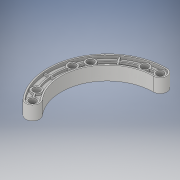
# Autodesk Inventor part: Curved_beam_6h
Saved by Autodesk Inventor 2019 (Build 230136000, 136)
## iProperties
Created: 2019-01-29
Part Number: Curved_beam_6h
Material: Generic
Document SubType Name: Modeling
Designer: Varga Daniel
Density: 1 g/cm^3
Appearance: Default
Author: Varga Daniel
Autodesk Inventor part; units mm, degrees
ref_plane "YZ Plane" through (0, 0, 0) normal (1, 0, 0) x (0, 1, 0)
ref_plane "XZ Plane" through (0, 0, 0) normal (0, 1, 0) x (-1, 0, 0)
ref_plane "XY Plane" through (0, 0, 0) normal (0, 0, 1) x (1, 0, 0)
derived "Base_part.ipt"
sketch "Sketch1" plane through (0, 0, 0) normal (0, 1, 0) x (-1, 0, 0)
  line L0 (5, 0) -> (25, 0)
  line L1 (30, 5) -> (30, 25)
  line L2 (25, 30) -> (5, 30)
  line L3 (0, 25) -> (0, 5)
  line L4 (5, 29) -> (25, 29)
  line L5 (29, 25) -> (29, 5)
  line L6 (25, 1) -> (5, 1)
  line L7 (1, 5) -> (1, 25)
  circle A0 centre (5, 5) radius 2.5
  circle A1 centre (5, 5) radius 3.5
  arc A2 (25, 0) -> (30, 5) centre (25, 5) ccw
  arc A3 (30, 25) -> (25, 30) centre (25, 25) ccw
  arc A4 (5, 30) -> (0, 25) centre (5, 25) ccw
  arc A5 (0, 5) -> (5, 0) centre (5, 5) ccw
  arc A6 (1, 5) -> (5, 1) centre (5, 5) ccw
  arc A7 (5, 29) -> (1, 25) centre (5, 25) ccw
  arc A8 (29, 25) -> (25, 29) centre (25, 25) ccw
  arc A9 (25, 1) -> (29, 5) centre (25, 5) ccw
  line L8 (49.1041, 15) -> (-27.081, 15) construction
  circle A10 centre (5, 15) radius 2.5
  circle A11 centre (5, 15) radius 3.5
  circle A12 centre (15, 5) radius 2.5
  circle A13 centre (15, 5) radius 3.5
  circle A14 centre (15, 15) radius 2.5
  circle A15 centre (15, 15) radius 3.5
  line L9 (1, 9.5) -> (1, 10.5)
  line L10 (29, 10.5) -> (29, 9.5)
  line L11 (31.1478, 10) -> (-2.4877, 10) construction
  line L12 (-2.8604, 5) -> (35.495, 5) construction
  line L13 (11.5359, 5.5) -> (8.4641, 5.5)
  line L14 (11.5359, 4.5) -> (8.4641, 4.5)
  line L15 (5, -2.5736) -> (5, 36.7522) construction
  line L16 (5.5, 8.4641) -> (5.5, 11.5359)
  line L17 (4.5, 8.4641) -> (4.5, 11.5359)
  line L18 (8.4641, 15.5) -> (11.5359, 15.5)
  line L19 (11.5359, 14.5) -> (8.4641, 14.5)
  line L20 (5.5, 1.5359) -> (5.5, 1)
  line L21 (4.5, 1.5359) -> (4.5, 1.0314)
  line L22 (1.5359, 4.5) -> (1.0314, 4.5)
  line L23 (1.5359, 5.5) -> (1, 5.5)
  line L24 (15, -1.4978) -> (15, 34.8784) construction
  line L25 (15.5, 8.4641) -> (15.5, 11.5359)
  line L26 (14.5, 11.5359) -> (14.5, 8.4641)
  line L27 (15.5, 1.5359) -> (15.5, 1)
  line L28 (14.5, 1.5359) -> (14.5, 1)
  line L29 (1.5359, 15.5) -> (1, 15.5)
  line L30 (1.5359, 14.5) -> (1, 14.5)
  line L31 (1, 10.5) -> (4.5, 10.5)
  line L32 (4.5, 10.5) -> (14.5, 10.5)
  line L33 (14.5, 9.5) -> (4.5, 9.5)
  line L34 (4.5, 9.5) -> (1, 9.5)
  line L35 (24.5, 8.4641) -> (24.5, 11.5359)
  line L36 (18.4641, 5.5) -> (21.5359, 5.5)
  line L37 (24.5, 10.5) -> (14.5, 10.5)
  line L38 (14.5, 9.5) -> (24.5, 9.5)
  circle A16 centre (25, 5) radius 2.5
  circle A17 centre (25, 5) radius 3.5
  line L39 (18.4641, 4.5) -> (21.5359, 4.5)
  line L40 (29, 9.5) -> (29, 10.5)
  line L41 (15.5, 11.5359) -> (15.5, 8.4641)
  line L42 (25.5, 8.4641) -> (25.5, 11.5359)
  line L43 (29, 10.5) -> (24.5, 10.5)
  line L44 (24.5, 9.5) -> (29, 9.5)
  line L45 (28.4641, 4.5) -> (28.9686, 4.5)
  line L46 (28.4641, 5.5) -> (29, 5.5)
  line L47 (15.5, 1.5359) -> (15.5, 1)
  line L48 (14.5, 1.5359) -> (14.5, 1)
  line L49 (24.5, 1.5359) -> (24.5, 1)
  line L50 (25.5, 1.5359) -> (25.5, 1.0314)
  line L51 (18.4641, 14.5) -> (21.5359, 14.5)
  line L52 (21.5359, 15.5) -> (18.4641, 15.5)
  circle A18 centre (25, 15) radius 2.5
  circle A19 centre (25, 15) radius 3.5
  line L53 (28.4641, 15.5) -> (29, 15.5)
  line L54 (28.4641, 14.5) -> (29, 14.5)
  line L55 (31.1478, 20) -> (-2.4877, 20) construction
  circle A20 centre (5, 25) radius 2.5
  circle A21 centre (5, 25) radius 3.5
  line L56 (15.5, 21.5359) -> (15.5, 18.4641)
  line L57 (15.5, 18.4641) -> (15.5, 21.5359)
  line L58 (14.5, 18.4641) -> (14.5, 21.5359)
  line L59 (24.5, 19.5) -> (14.5, 19.5)
  line L60 (15.5, 20.5) -> (25.5, 20.5)
  circle A22 centre (15, 25) radius 2.5
  circle A23 centre (15, 25) radius 3.5
  line L61 (11.5359, 25.5) -> (8.4641, 25.5)
  line L62 (11.5359, 24.5) -> (8.4641, 24.5)
  line L63 (4.5, 19.5) -> (14.5, 19.5)
  line L64 (15.5, 20.5) -> (5.5, 20.5)
  line L65 (18.4641, 24.5) -> (21.5359, 24.5)
  line L66 (18.4641, 25.5) -> (21.5359, 25.5)
  line L67 (15.5, 28.4641) -> (15.5, 29)
  line L68 (15.5, 28.4641) -> (15.5, 29)
  line L69 (14.5, 28.4641) -> (14.5, 29)
  line L70 (14.5, 28.4641) -> (14.5, 29)
  line L71 (1, 20.5) -> (1, 19.5)
  line L72 (5.5, 21.5359) -> (5.5, 18.4641)
  line L73 (4.5, 21.5359) -> (4.5, 18.4641)
  line L74 (1, 19.5) -> (4.5, 19.5)
  line L75 (5.5, 20.5) -> (1, 20.5)
  line L76 (5.5, 28.4641) -> (5.5, 29)
  line L77 (4.5, 28.4641) -> (4.5, 28.9686)
  line L78 (1.5359, 25.5) -> (1.0314, 25.5)
  line L79 (1.5359, 24.5) -> (1, 24.5)
  line L80 (24.5, 21.5359) -> (24.5, 18.4641)
  line L81 (29, 19.5) -> (29, 20.5)
  circle A24 centre (25, 25) radius 2.5
  circle A25 centre (25, 25) radius 3.5
  line L82 (24.5, 28.4641) -> (24.5, 29)
  line L83 (25.5, 28.4641) -> (25.5, 28.9686)
  line L84 (28.4641, 25.5) -> (28.9686, 25.5)
  line L85 (25.5, 21.5359) -> (25.5, 18.4641)
  line L86 (28.4641, 24.5) -> (29, 24.5)
  line L87 (25.5, 20.5) -> (29, 20.5)
  line L88 (29, 19.5) -> (24.5, 19.5)
  line L89 (29, 20.5) -> (29, 19.5)
  point P0 (0, 0)
  point P1 (30, 30)
  point P2 (0, 30)
  point P3 (5, 15)
  point P4 (5, 15)
  point P5 (15, 5)
  point P6 (15, 15)
  point P7 (5.5, 10.5)
  point P8 (5.5, 9.5)
  point P9 (14.5, 11.5359)
  point P10 (15.5, 10.5)
  point P11 (15.5, 9.5)
  point P12 (25, 5)
  point P13 (25, 5)
  point P14 (30, 0)
  point P15 (25.5, 9.5)
  point P16 (25.5, 10.5)
  point P17 (25, 15)
  point P18 (25, 15)
  point P19 (15, 25)
  point P20 (-2.8604, 25)
  point P21 (25, 25)
  point P22 (5, 25)
  point P23 (5, 25)
  point P24 (25, 25)
  point P25 (15.5, 19.5)
  point P26 (14.5, 18.4641)
  point P27 (24.5, 20.5)
  point P28 (15, 31.4978)
  point P29 (5, 32.5736)
  point P30 (5.5, 19.5)
  point P31 (14.5, 20.5)
  point P32 (4.5, 20.5)
  point P33 (25, 25)
  point P34 (25, 25)
  point P35 (25.5, 19.5)
sketch "Sketch2" plane through (0, 0, 0) normal (0, 1, 0) x (-1, 0, 0)
  arc A0 (0, -33.5) -> (25.3746, 21.8719) centre (0, 0) ccw
  arc A1 (0, -38.5) -> (29.1618, 25.1364) centre (0, 0) ccw construction
  arc A2 (0, -43.5) -> (32.9491, 28.4008) centre (0, 0) ccw
  line L0 (0, -33.5) -> (0, -43.5) construction
  line L1 (25.3746, 21.8719) -> (32.9491, 28.4008) construction
  arc A3 (0, -34.5) -> (26.132, 22.5248) centre (0, 0) ccw
  arc A4 (0, -42.5) -> (32.1916, 27.7479) centre (0, 0) ccw
  circle A5 centre (0, -38.5) radius 3.5
  circle A6 centre (9.9153, -37.2013) radius 3.5
  arc A7 (0, -33.5) -> (0, -43.5) centre (0, -38.5) ccw
  arc A8 (0, -34.5) -> (0, -42.5) centre (0, -38.5) ccw
  arc A9 (32.9491, 28.4008) -> (25.3746, 21.8719) centre (29.1618, 25.1364) ccw
  arc A10 (32.1916, 27.7479) -> (26.132, 22.5248) centre (29.1618, 25.1364) ccw
  circle A11 centre (29.1618, 25.1364) radius 3.5
  circle A12 centre (34.6518, 16.7781) radius 3.5
  circle A13 centre (32.6206, -20.4486) radius 3.5
  circle A14 centre (36.7866, -11.3577) radius 3.5
  line L2 (0, 0) -> (39.5455, -18.122) construction
  arc A15 (27.1485, 27.9993) -> (26.7812, 28.3508) centre (0, 0) ccw
  arc A16 (26.4204, 27.3123) -> (26.0574, 27.6588) centre (0, 0) ccw
  arc A17 (32.5632, 19.5866) -> (30.9097, 22.1041) centre (0, 0) ccw
  arc A18 (33.4436, 20.063) -> (31.6966, 22.7228) centre (0, 0) ccw
  arc A19 (38.1429, -8.1312) -> (36.4794, 13.7932) centre (0, 0) ccw
  arc A20 (37.1741, -7.8793) -> (35.5597, 13.3979) centre (0, 0) ccw
  arc A21 (33.8909, -17.1873) -> (35.1457, -14.4492) centre (0, 0) ccw
  arc A22 (34.7622, -17.6803) -> (36.0879, -14.7873) centre (0, 0) ccw
  arc A23 (13.0684, -35.6822) -> (30.2389, -23.0133) centre (0, 0) ccw
  arc A24 (13.3695, -36.6368) -> (31.0622, -23.5826) centre (0, 0) ccw
  arc A25 (-3.9375, -37.7955) -> (-3.438, -37.8442) centre (0, 0) ccw
  arc A26 (3.438, -37.8442) -> (6.4244, -37.453) centre (0, 0) ccw
  arc A27 (-3.9891, -38.7955) -> (-3.483, -38.8442) centre (0, 0) ccw
  arc A28 (3.483, -38.8442) -> (6.6384, -38.4309) centre (0, 0) ccw
  line L3 (0, -38.5) -> (0, 0) construction
  line L4 (9.9153, -37.2013) -> (0, 0) construction
  line L5 (32.6206, -20.4486) -> (0, 0) construction
  line L6 (36.7866, -11.3577) -> (0, 0) construction
  line L7 (34.6518, 16.7781) -> (0, 0) construction
  line L8 (29.1618, 25.1364) -> (0, 0) construction
  line L9 (8.4011, -33.4615) -> (8.54, -33.9828)
  line L10 (10.3243, -40.6773) -> (10.4616, -41.1923)
  line L11 (9.3673, -33.204) -> (9.5063, -33.7253)
  line L12 (11.2906, -40.4198) -> (11.4278, -40.9348)
  line L13 (0.5, -34.4964) -> (0.5, -35.0359)
  line L14 (0.5, -41.9641) -> (0.5, -42.4971)
  line L15 (-0.5, -42.4686) -> (-0.5, -41.9641)
  line L16 (-0.5, -35.0359) -> (-0.5, -34.5314)
  circle A29 centre (0, -38.5) radius 2.5
  circle A30 centre (15, 5) radius 2.5 construction
  circle A31 centre (15, 5) radius 3.5 construction
  line L17 (18.4641, 5.5) -> (21.5359, 5.5) construction
  line L18 (-2.8604, 5) -> (35.495, 5) construction
  line L19 (18.4641, 4.5) -> (21.5359, 4.5) construction
  line L20 (1, 5) -> (1, 25) construction
  line L21 (0, 25) -> (0, 5) construction
  circle A32 centre (9.9153, -37.2013) radius 2.5
  circle A33 centre (32.6206, -20.4486) radius 2.5
  circle A34 centre (36.7866, -11.3577) radius 2.5
  circle A35 centre (34.6518, 16.7781) radius 2.5
  circle A36 centre (29.1618, 25.1364) radius 2.5
  line L22 (28.9628, -18.7458) -> (29.4199, -19.0324)
  line L23 (36.2728, -22.148) -> (35.8213, -21.8649)
  line L24 (29.9511, -18.1851) -> (29.4939, -17.8985)
  line L25 (35.2901, -22.7122) -> (35.7417, -22.9953)
  line L26 (32.8136, -10.6544) -> (33.3291, -10.8135)
  line L27 (39.949, -12.8574) -> (40.4582, -13.0146)
  line L28 (40.7532, -12.0591) -> (40.244, -11.9019)
  line L29 (33.6241, -9.858) -> (33.1086, -9.6989)
  line L30 (31.2662, 14.5833) -> (31.7518, 14.8184)
  line L31 (37.9875, 17.8377) -> (38.4672, 18.07)
  line L32 (30.8304, 15.4834) -> (31.316, 15.7185)
  line L33 (37.5517, 18.7378) -> (38.0314, 18.97)
  line L34 (31.8414, 28.1062) -> (31.4593, 27.7768)
  line L35 (26.2115, 23.2534) -> (25.8294, 22.924)
  line L36 (26.4557, 22.1437) -> (26.8644, 22.496)
  line L37 (32.1122, 27.0193) -> (32.5159, 27.3673)
  line L38 (38.3897, 2.9128) -> (0, 0) construction
  line L39 (42.3374, 3.7138) -> (38.8472, 3.449)
  line L40 (37.85, 3.3733) -> (34.3597, 3.1085)
  line L41 (34.4353, 2.1113) -> (37.9256, 2.3762)
  line L42 (38.9229, 2.4518) -> (42.4131, 2.7166)
  line L43 (20.8833, -27.4615) -> (22.9615, -30.2782)
  line L44 (23.5553, -31.0829) -> (25.6335, -33.8995)
  line L45 (20.0787, -28.0553) -> (22.1569, -30.8719)
  line L46 (22.7506, -31.6766) -> (24.8288, -34.4932)
  line L47 (25.2329, -34.1987) -> (0, 0) construction
  dimension "d7" = 7
  dimension "d8" = 7
  dimension "d16" = 7
  dimension "d17" = 7
  dimension "d22" = 7
  dimension "d23" = 7
  dimension "d0" = 33.5
  dimension "d3" = 10
  dimension "d4" = 5
  dimension "d5" = 1
  dimension "d6" = 1
  dimension "d14" = 10
  dimension "d15" = 4
  dimension "d21" = 10
  dimension "d24" = 10
  dimension "d28" = 5
  dimension "d29" = 70
  dimension "d34" = 1
  dimension "d35" = 0.5
  dimension "d37" = 1
  dimension "d38" = 1
  dimension "d39" = 5
  dimension "d40" = 5
  dimension "d41" = 7
  dimension "d42" = 5
  dimension "d43" = 5
  dimension "d44" = 5
  dimension "d45" = 5
  dimension "d46" = 5
  dimension "d48" = 1
  dimension "d49" = 1
  dimension "d51" = 1
  dimension "d53" = 1
  dimension "d54" = 42.994
  dimension "d55" = 21.497
  dimension "d57" = 1
  dimension "d74" = 1
  constraints: 86 end point, 66 point on circle, 27 centre point, 27 parallel, 16 collinear, 14 coincident, 12 concentric, 7 point on line, 2 midpoint, 2 vertical, 1 tangent, 111 other
  measures "d0" radius of A0
  measures "d3" radial gap between concentric circles of A2 A0
  measures "d4" radial gap between concentric circles of A1 A0
  measures "d14" distance of A1.start L4.start
  measures "d15" radius of A8
  measures "d21" distance of A9.centre L7.start
  measures "d24" distance of L5.start L6.start
  measures "d28" distance from line of L6.start L2
  measures "d29" distance of A1.end A1.start
  measures "d34" radial gap between concentric circles of A26 A28
  measures "d35" radial gap between concentric circles of A1 A28
  measures "d37" distance between parallel lines of L16 L13
  measures "d38" distance between parallel lines of L9 L11
  measures "d39" diameter of A29
  measures "d40" diameter of A30
  measures "d41" diameter of A31
  measures "d42" diameter of A32
  measures "d43" diameter of A33
  measures "d44" diameter of A34
  measures "d45" diameter of A35
  measures "d46" diameter of A36
  measures "d48" distance between parallel lines of L24 L22
  measures "d49" distance between parallel lines of L29 L26
  measures "d51" distance between parallel lines of L32 L30
  measures "d53" distance between parallel lines of L35 L36
  measures "d54" angle of L7 L6
  measures "d55" angle of L38 L6
  measures "d57" distance between parallel lines of L40 L41
  measures "d74" distance of L45.start L43.start
extrude "Extrusion1" add sketch "Sketch2" along normal blind 5 contours A0 A9 A2 A7
extrude "Extrusion2" add sketch "Sketch2" against normal blind 5 contours A0 A9 A2 A7
extrude "Extrusion3" add sketch "Sketch2" along normal blind 4.2 contours A3 L13 A5 L16 A8 | A3 L11 A6 L9 | A5 | A25 A5 A27 A8 | A6 | A26 A6 A28 A5 | A3 L43 A23 L45 | L15 A5 L14 A4 A8 | A23 A13 A24 A6 | A3 L24 A13 L22 | A6 L12 A4 L10 | A13 | A24 L44 A4 L46 | A3 L29 A14 L26 | A14 | A21 A14 A22 A13 | A13 L23 A4 L25 | A3 L40 A20 L41 | A20 A12 A19 A14 | A3 L32 A12 L30 | A14 L28 A4 L27 | A12 | A19 L39 A4 L42 | A3 A10 L35 A11 L36 | A11 | A17 A11 A18 A12 | A12 L33 A4 L31 | A10 A15 A11 A16 | L37 A11 L34 A10 A4
extrude "Extrusion4" add sketch "Sketch2" against normal blind 4.2 contours A3 L13 A5 L16 A8 | A3 L11 A6 L9 | A5 | A25 A5 A27 A8 | A6 | A26 A6 A28 A5 | A3 L43 A23 L45 | L15 A5 L14 A4 A8 | A23 A13 A24 A6 | A3 L24 A13 L22 | A6 L12 A4 L10 | A13 | A24 L44 A4 L46 | A3 L29 A14 L26 | A14 | A21 A14 A22 A13 | A13 L23 A4 L25 | A3 L40 A20 L41 | A20 A12 A19 A14 | A3 L32 A12 L30 | A14 L28 A4 L27 | A12 | A19 L39 A4 L42 | A3 A10 L35 A11 L36 | A11 | A17 A11 A18 A12 | A12 L33 A4 L31 | A10 A15 A11 A16 | L37 A11 L34 A10 A4
extrude "Extrusion5" add sketch "Sketch2" along normal blind 2.7 contours A3 L9 A6 A26 A5 L13 | L16 A5 A25 A8 | A3 L45 A23 A6 L11 | A27 A5 L15 A8 | A3 L22 A13 A23 L43 | A6 L10 A4 L14 A5 A28 | A24 L46 A4 L12 A6 | A3 L26 A14 A21 A13 L24 | A13 L25 A4 L44 A24 | A3 L41 A20 A14 L29 | A22 A14 L27 A4 L23 A13 | A3 L30 A12 A20 L40 | A19 L42 A4 L28 A14 | A3 L36 A11 A17 A12 L32 | A12 L31 A4 L39 A19 | A10 A16 A11 L35 | A18 A11 L37 A4 L33 A12 | A10 L34 A11 A15
extrude "Extrusion6" add sketch "Sketch2" against normal blind 2.7 contours A3 L9 A6 A26 A5 L13 | L16 A5 A25 A8 | A3 L45 A23 A6 L11 | A27 A5 L15 A8 | A3 L22 A13 A23 L43 | A6 L10 A4 L14 A5 A28 | A24 L46 A4 L12 A6 | A3 L26 A14 A21 A13 L24 | A13 L25 A4 L44 A24 | A3 L41 A20 A14 L29 | A22 A14 L27 A4 L23 A13 | A3 L30 A12 A20 L40 | A19 L42 A4 L28 A14 | A3 L36 A11 A17 A12 L32 | A12 L31 A4 L39 A19 | A10 A16 A11 L35 | A18 A11 L37 A4 L33 A12 | A10 L34 A11 A15
equation "\"d7\" = d41"
equation "\"d8\" = d7"
equation "\"d16\" = d7"
equation "\"d17\" = d7"
equation "\"d22\" = d7"
equation "\"d23\" = d7"
equation "\"d4\" = 0.5 * d3"
equation "\"d5\" = Wall_thickness"
equation "\"d6\" = Wall_thickness"
equation "\"d28\" = 0.5 * d24"
equation "\"d34\" = Inner_route_thickness"
equation "\"d35\" = 0.5 * d34"
equation "\"d37\" = Inner_route_thickness"
equation "\"d38\" = d37"
equation "\"d39\" = d40"
equation "\"d42\" = d39"
equation "\"d43\" = d39"
equation "\"d44\" = d39"
equation "\"d45\" = d39"
equation "\"d46\" = d39"
equation "\"d48\" = d37"
equation "\"d49\" = d37"
equation "\"d30\" = Inner_route_thickness"
equation "\"d31\" = 0.5 * d30"
equation "\"d32\" = Inner_route_thickness"
equation "\"d33\" = 0.5 * d32"
equation "\"d47\" = d37"
equation "\"Wall_thickness\" = 1"
equation "\"Inner_route_thickness\" = 1"
body "Solid1"
